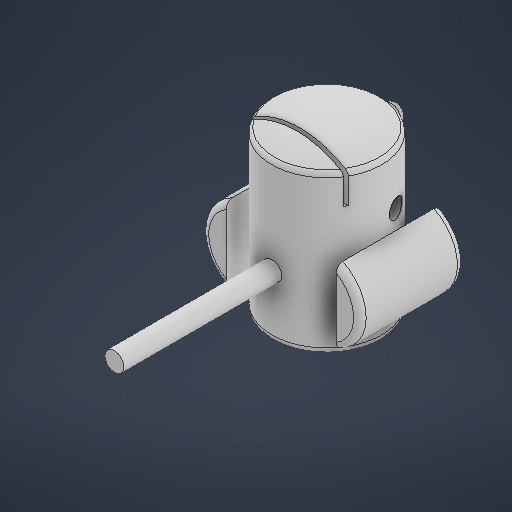
# Autodesk Inventor part: součást 4
Saved by Autodesk Inventor 2025.1 (Build 291241000, 241)
## iProperties
Created: 2025-04-28
Part Number: součást 4
Material: Všeobecné
Document SubType Name: Modeling
Designer: Dominik Petříček
Density: 1 g/cm^3
Appearance: Výchozí
Author: Dominik Petříček
Autodesk Inventor part; units mm, degrees
sketch "Náčrt1" plane through (0, 0, 0) normal (0, 0, 1) x (1, 0, 0)
  line L0 (0, 0) -> (0, -59)
  line L1 (0, -59) -> (0, -19)
  arc A0 (-16.3158, -55.5212) -> (0, -59) centre (0, -19) ccw
  line L2 (0, -59) -> (0, -29.5)
  line L3 (-17.5, -29.5) -> (-17.5, -53.6951)
  line L4 (-17.5, -29.5) -> (6.6951, -29.5) construction
  line L5 (-17.5, -29.5) -> (-17.5, -6.8923)
  line L6 (0, 0) -> (0, -29)
  arc A1 (0, 0) -> (-16.6481, -5.2547) centre (0, -29) ccw
  line L7 (-17.5, -7) -> (-17.5, -6.8923)
  arc A2 (-16.6481, -5.2547) -> (-17.5, -6.8923) centre (-15.5, -6.8923) ccw
  arc A3 (-17.5, -53.6951) -> (-16.3158, -55.5212) centre (-15.5, -53.6951) ccw
  dimension "d79" = 59
  dimension "d80" = 40
  dimension "d81" = 29.5
  dimension "d82" = 17.5
  dimension "d84" = 90
  dimension "d85" = 22.5
  dimension "d86" = 29
  dimension "d89" = 2
  dimension "d90" = 2
  constraints: 16 end point, 8 point on circle, 4 centre point, 4 point on line, 4 tangent, 4 vertical, 2 coincident, 1 horizontal, 1 perpendicular
  measures "d79" distance of L0.start L0.end
  measures "d80" distance of L0.end L1.end
  measures "d81" distance of L0.end L2.end
  measures "d82" distance of L2.end L3.start
  measures "d84" angle of L3 L4
  measures "d85" distance of L3.start L7.start
  measures "d86" distance of L0.start L6.end
  measures "d89" radius of A2
  measures "d90" radius of A3
revolve "Rotace1" add sketch "Náčrt1" angle 360 about axis through (0, 0, 0) along (0, -1, 0)
ref_plane "Pracovní rovina1" through (17.5, 0, 0) normal (1, 0, 0) x (0, 1, 0)
sketch "Náčrt2" plane through (17.5, 0, 0) normal (1, 0, 0) x (0, 1, 0)
  line L0 (0, 0) -> (-22, 0)
  line L1 (-6.8923, 17.5) -> (-6.8923, -17.5) projected
  line L2 (-6.8923, -17.5) -> (-6.8923, -5.5)
  line L3 (-6.8923, -5.5) -> (-22, -5.5)
  circle A0 centre (-22, -5.5) radius 3
  line L4 (-6.8923, 17.5) -> (-6.8923, 9.5)
  line L5 (0, 0) -> (-15, 0)
  line L6 (-15, 0) -> (-15, 9.5)
  line L7 (-15, 9.5) -> (-1.6002, 9.5)
  arc A1 (-5.2547, -16.6481) -> (-5.2547, 16.6481) centre (-29, 0) ccw projected
  line L8 (-15, 9.5) -> (-15, 8.5)
  line L9 (-15, 8.5) -> (-1.2737, 8.5)
  line L10 (-5.2547, 16.6481) -> (-5.2547, -16.6481) projected
  arc A2 (-55.5212, 16.3158) -> (-55.5212, -16.3158) centre (-19, 0) ccw projected
  dimension "d9" = 22
  dimension "d10" = 12
  dimension "d11" = 6
  dimension "d12" = 8
  dimension "d13" = 15
  dimension "d14" = 1
  constraints: 18 end point, 4 point on line, 3 perpendicular, 2 point on circle, 1 centre point, 1 coincident, 1 horizontal, 1 parallel
  measures "d9" distance of L0.start L0.end
  measures "d10" distance of L1.end L2.end
  measures "d11" diameter of A0
  measures "d12" distance of L1.start L4.end
  measures "d13" distance of L0.start L5.end
  measures "d14" distance of L6.end L8.end
extrude "Vysunutí1" cut sketch "Náčrt2" against normal through all contours L9 L10 L7 A1 | L9 L1 L7 L10 | L9 L6 L7 L1 | A0
sketch "Náčrt3" plane through (0, 0, 0) normal (1, 0, 0) x (0, 1, 0)
  line L0 (0, 0) -> (-12, 0)
  line L1 (0, 0) -> (12, 0) construction
  line L2 (-12, 0) -> (-12, -17.5)
  line L3 (-6.8923, -17.5) -> (-53.6951, -17.5) projected
  line L4 (-12, -17.5) -> (-9, -17.5)
  line L5 (-12, -17.5) -> (-15, -17.5)
  line L6 (-15, -17.5) -> (-15, -20.5)
  line L7 (-9, -17.5) -> (-9, -20.5)
  line L8 (-11, -22.5) -> (-13, -22.5)
  arc A0 (-11, -22.5) -> (-9, -20.5) centre (-11, -20.5) ccw
  arc A1 (-15, -20.5) -> (-13, -22.5) centre (-13, -20.5) ccw
  line L9 (-9, -17.5) -> (-9, -14.1707)
  line L10 (-9, -14.1707) -> (-15, -14.1707)
  line L11 (-15, -14.1707) -> (-15, -17.5)
  line L12 (-9, -17.5) -> (-15, -17.5)
  line L13 (-12, -14.1707) -> (-12, -22.5)
  point P0 (-15, -22.5)
  point P1 (-9, -22.5)
  dimension "d20" = 12
  dimension "d21" = 180
  dimension "d22" = 3
  dimension "d23" = 3
  dimension "d24" = 5
  dimension "d25" = 5
  dimension "d26" = 2
  constraints: 26 end point, 7 point on line, 5 perpendicular, 4 point on circle, 4 tangent, 2 centre point, 2 horizontal, 2 midpoint, 2 vertical, 1 collinear, 1 equal radius
  measures "d20" distance of L0.start L0.end
  measures "d21" angle of L0 L1
  measures "d22" distance of L2.end L4.end
  measures "d23" distance of L2.end L5.end
  measures "d24" distance of L5.end point (-15, -22.5)
  measures "d25" distance of L4.end point (-9, -22.5)
  measures "d26" radius of A0
revolve "Rotace2" add sketch "Náčrt3" angle 360 about axis through (0, -12, -14.1707) along (0, 0, -1) contours L10 L9 L3 L2 | L3 L7 A0 L8 L13
sketch "Náčrt4" plane through (0, 0, 0) normal (0, 0, 1) x (1, 0, 0)
  arc A0 (-16.3158, -55.5212) -> (16.3158, -55.5212) centre (0, -19) ccw projected
  line L0 (0, -59) -> (0, -36)
  circle A1 centre (0, -36) radius 3
  point P0 (0, 0)
  dimension "d28" = 23
  dimension "d29" = 6
  constraints: 2 end point, 1 centre point, 1 coincident, 1 point on circle, 1 vertical
  measures "d28" distance of L0.start L0.end
  measures "d29" diameter of A1
extrude "Vysunutí2" add sketch "Náčrt4" along normal blind 67.5
ref_plane "Pracovní rovina3" through (0, -59, 0) normal (0, 1, 0) x (-1, 0, 0)
sketch "Náčrt5" plane through (0, -59, 0) normal (0, 1, 0) x (-1, 0, 0)
  line L0 (0, 0) -> (-17.5, 0)
  circle A0 centre (0, 0) radius 17.5 projected
  line L1 (-17.5, 0) -> (-17.5, 14.5)
  line L2 (-17.5, 14.5) -> (-17.5, -18.5)
  line L3 (-17.5, -18.5) -> (-23, -18.5)
  line L4 (-25, -16.5) -> (-25, 12.5)
  line L5 (-23, 14.5) -> (-17.5, 14.5)
  line L6 (-25, 12.5) -> (-25, 14.5)
  line L7 (-25, 14.5) -> (-23, 14.5)
  line L8 (-25, -16.5) -> (-25, -18.5)
  line L9 (-25, -18.5) -> (-23, -18.5)
  dimension "d32" = 14.5
  dimension "d33" = 33
  dimension "d34" = 7.5
  constraints: 20 end point, 7 perpendicular, 3 point on line, 1 horizontal, 1 horizontal alignment, 1 vertical, 1 other
  measures "d32" distance of L0.end L1.end
  measures "d33" distance of L1.end L2.end
  measures "d34" distance of L2.end L8.end
extrude "Vysunutí3" add sketch "Náčrt5" along normal blind 32 contours L2 L3 L9 L8 L4 L6 L7 L5 L1
ref_plane "Pracovní rovina4" through (23, -59, -18.5) normal (0, 0, -1) x (-1, 0, 0)
sketch "Náčrt6" plane through (23, -59, -18.5) normal (0, 0, -1) x (-1, 0, 0)
  arc A0 (6.6842, 3.4788) -> (39.3158, 3.4788) centre (23, 40) ccw projected
  line L0 (23, 0) -> (23, 20)
  line L1 (23, 20) -> (-2, 20)
  line L2 (-2, 0) -> (-2, 32) projected
  line L3 (-2, 20) -> (-2, 8)
  line L4 (-2, 20) -> (11, 20)
  circle A1 centre (11, 20) radius 13
  line L5 (-2, 0) -> (0, 0) projected
  line L6 (0, 0) -> (0, 32) projected
  line L7 (-2, 32) -> (0, 32) projected
  line L8 (-2, 0) -> (-2, 32) projected
  line L9 (-2, 0) -> (5.5, 0) projected
  line L10 (5.5, 0) -> (5.5, 32) projected
  line L11 (-2, 32) -> (5.5, 32) projected
  line L12 (-2, 0) -> (-2, 32) projected
  point P0 (23, 59)
  point P1 (5.5, 31.7792)
  point P2 (5.5, 8.2208)
  dimension "d38" = 20
  dimension "d39" = 12
  dimension "d40" = 13
  constraints: 8 end point, 3 point on line, 1 coincident, 1 horizontal, 1 point on circle, 1 vertical, 3 other
  measures "d38" distance of L0.start L0.end
  measures "d39" distance of L1.end L3.end
  measures "d40" distance of L1.end L4.end
extrude "Vysunutí4" cut sketch "Náčrt6" against normal through all contours L10 L9 L6 A1 | L6 L5 L2 A1 | A1 L6 L11 L10 | L2 L7 L6 A1
fillet "Zaoblení3" radius 2 2 edges at (25, -39, -18.5) (25, -39, 14.5)
mirror "Zrcadlit2" about plane through (0, 0, 0) normal (1, 0, 0) of "Zaoblení3", "Vysunutí4", "Vysunutí3"
